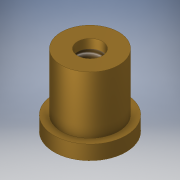
# Autodesk Inventor part: feet type 2 part 1
Saved by Autodesk Inventor 2018 (Build 220112000, 112)
## iProperties
Created: 2018-10-16
Part Number: feet type 2 part 1
Material: Brass, Soft Yellow
Document SubType Name: Modeling
Designer: freyja
Density: 8.47 g/cm^3
Appearance: Brass - Satin
Mass: 3.4022 g
Surface Area: 4.63612 cm^2
Volume: 0.401676 cm^3
Author: freyja
Autodesk Inventor part; units mm, degrees
ref_plane "YZ Plane" through (0, 0, 0) normal (1, 0, 0) x (0, 1, 0)
ref_plane "XZ Plane" through (0, 0, 0) normal (0, 1, 0) x (-1, 0, 0)
ref_plane "XY Plane" through (0, 0, 0) normal (0, 0, 1) x (1, 0, 0)
sketch "Sketch1" plane through (0, 0, 0) normal (0, 1, 0) x (-1, 0, 0)
  circle A0 centre (0, 0) radius 4.7625
  dimension "d0" = 9.525
  constraints: 1 centre point, 1 coincident
  measures "d0" diameter of A0
extrude "Extrusion1" add sketch "Sketch1" along normal blind 9.525
sketch "Sketch2" plane through (0, 9.525, 0) normal (0, 1, 0) x (1, 0, 0)
  circle A0 centre (0, 0) radius 6.35
  circle A1 centre (0, 0) radius 3.81
  dimension "d3" = 12.7
  dimension "d4" = 7.62
  constraints: 2 centre point, 2 coincident
  measures "d3" diameter of A0
  measures "d4" diameter of A1
extrude "Extrusion2" cut sketch "Sketch2" against normal blind 7.62
sketch "Sketch3" plane through (0, 0, 0) normal (0, -1, 0) x (1, 0, 0)
  circle A0 centre (0, 0) radius 1.5777
  constraints: 1 centre point, 1 coincident
hole "Hole1" at (0, 0, 0) direction (0, 1, 0) diameter 3.302 end through all thread size "8-32 UNC" class "2B" standard "ANSI Unified Screw Threads"
body "Solid1"
